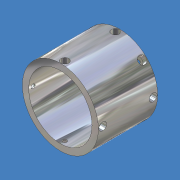
# Autodesk Inventor part: BB2-RingGear
Saved by Autodesk Inventor 2012 (Build 160160000, 160)
## iProperties
Company: FirstCadLibrary
Shininess: 64.0
Length Units: 11269
Angle Units: 11279
Time Units: 11290
Mass Units: 11283
Length Display Precision: 3
Angle Display Precision: 2
Compacted: True
Part Number: BB2-RingGear
Document SubType Name: Modeling
Created: 2007-01-08
Designer: Ed Sparks
Material: Steel, Mild
Catalog Web Link: www.banebots.com
Vendor: BaneBots
Mass: 305.369 g
Surface Area: 187.722 cm^2
Volume: 38.851 cm^3
Density: 7.86 g/cm^3
Density: 0.0
Volumn: 0.0
Area: 0.0
PropertySet Name: Model Information
Control State: 0
Master: False
Checked Out: False
Author: Ed Sparks
Autodesk Inventor part; units mm, degrees
ref_plane "YZ Plane" through (0, 0, 0) normal (1, 0, 0) x (0, 1, 0)
ref_plane "XZ Plane" through (0, 0, 0) normal (0, 1, 0) x (-1, 0, 0)
sketch "Sketch1" plane through (0, 0, 0) normal (0, 0, 1) x (1, 0, 0)
  circle A0 centre (0, 0) radius 25
  circle A1 centre (0, 0) radius 30
  dimension "d0" = 50
  dimension "d1" = 60
  constraints: 2 centre point, 2 coincident, 1 concentric, 1 other
  measures "d0" diameter of A0
  measures "d1" diameter of A1
extrude "Extrusion1" add sketch "Sketch1" along normal blind 46.8
ref_plane "Work Plane1" through (-30, 0, 0) normal (1, 0, 0) x (0, 1, 0)
sketch "Sketch3" plane through (-30, 0, 0) normal (1, 0, 0) x (0, 1, 0)
  line L0 (-30, 0) -> (30, 0) projected
  line L1 (0, 0) -> (0, 28.195) construction
  point P0 (0, 3.5)
  dimension "d5" = 3.5
  constraints: 2 end point, 1 midpoint, 1 perpendicular, 1 point on line
  measures "d5" distance from line of L0 point (0, 3.5)
hole "Hole1" at (-30, 0, 3.5) direction (1, 0, 0) diameter 3.2 depth 8 tip angle 118 counterbore diameter 6.2 counterbore depth 4.2
pattern_circular "Circular Pattern1" count 8 over 360 about axis through (0, 0, 0) along (0, 0, 1) of "Hole1"
sketch "Sketch4" plane through (-30, 0, 0) normal (1, 0, 0) x (0, 1, 0)
  line L0 (-30, 46.8) -> (30, 46.8) projected
  line L1 (0, 46.8) -> (0, 26.1397) construction
  point P0 (0, 43.3)
  dimension "d16" = 3.5
  constraints: 2 end point, 1 midpoint, 1 perpendicular, 1 point on line
  measures "d16" distance from line of L0 point (0, 43.3)
hole "Hole2" at (-30, 0, 43.3) direction (1, 0, 0) diameter 3.2 depth 8 tip angle 118 counterbore diameter 6.2 counterbore depth 4.2
pattern_circular "Circular Pattern2" count 4 over 360 about axis through (0, 0, 0) along (0, 0, 1) of "Hole2"
body "Solid1"
